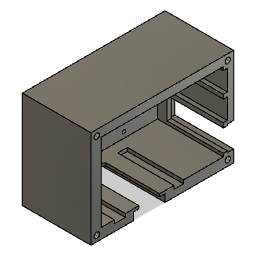
Main Pi Case v10 (Autodesk Fusion 360 design; units mm, degrees)
Autodesk Fusion 360 part; units mm, degrees
sketch "Sketch1" plane through (0, 0, 0) normal (1, 0, 0) x (0, 0, -1)
  line L0 (-44.5, 28) -> (44.5, 28)
  line L1 (44.5, 28) -> (44.5, -28)
  line L2 (44.5, -28) -> (-44.5, -28)
  line L3 (-44.5, -28) -> (-44.5, 28)
  line L4 (-44.5, 28) -> (44.5, -28) construction
  line L5 (44.5, 28) -> (-44.5, -28) construction
  circle A0 centre (-38, 24.5) radius 1.25
  circle A1 centre (-38, -24.5) radius 1.25
  circle A2 centre (20, 25.1038) radius 1.25
  circle A3 centre (20, -23.8962) radius 1.25
  line L6 (-52, 35.5) -> (52, 35.5)
  line L7 (52, 35.5) -> (52, -35.5)
  line L8 (52, -35.5) -> (-52, -35.5)
  line L9 (-52, -35.5) -> (-52, 35.5)
  line L10 (-52, 35.5) -> (52, -35.5) construction
  line L11 (52, 35.5) -> (-52, -35.5) construction
  line L12 (-44.5, 28) -> (-44.5, 29)
  line L13 (-44.5, 29) -> (44.5, 29)
  line L14 (44.5, 29) -> (44.5, 28)
  circle A4 centre (0, 0) radius 13.5
  line L15 (-15, 15) -> (15, 15)
  line L16 (15, 15) -> (15, -15)
  line L17 (15, -15) -> (-15, -15)
  line L18 (-15, -15) -> (-15, 15)
  line L19 (-15, 15) -> (15, -15) construction
  line L20 (15, 15) -> (-15, -15) construction
  circle A5 centre (13, 13) radius 1.5
  circle A6 centre (-13, 13) radius 1.5
  circle A7 centre (-13, -13) radius 1.5
  circle A8 centre (13, -13) radius 1.5
  dimension "d1" = 89
  dimension "d2" = 56
  dimension "d3" = 2.5
  dimension "d4" = 3.5
  dimension "d5" = 6.5
  dimension "d6" = 2.5
  dimension "d7" = 6.5
  dimension "d8" = 49
  dimension "d9" = 2.5
  dimension "d10" = 2.5
  dimension "d11" = 49
  dimension "d12" = 58
  dimension "d13" = 58
  dimension "d16" = 104
  dimension "d17" = 71
  dimension "d86" = 27
  dimension "d87" = 30
  dimension "d88" = 30
  dimension "d89" = 3
  dimension "d90" = 3
  dimension "d91" = 3
  dimension "d92" = 3
  dimension "d93" = 2
  dimension "d94" = 2
  dimension "d95" = 2
  dimension "d96" = 2
  constraint horizontal L0
  constraint perpendicular L0 L1
  constraint parallel L0 L2
  constraint parallel L1 L3
  constraint coincident L4 A4.centre
  constraint coincident L5 A4.centre
  constraint coincident A4.centre origin
  constraint horizontal L6
  constraint perpendicular L6 L7
  constraint parallel L6 L8
  constraint parallel L7 L9
  constraint coincident L10 A4.centre
  constraint coincident L11 A4.centre
  constraint perpendicular L0 L12
  constraint perpendicular L12 L13
  constraint perpendicular L0 L14
  constraint horizontal L15
  constraint perpendicular L15 L16
  constraint parallel L15 L17
  constraint parallel L16 L18
  constraint coincident L19 A4.centre
  constraint coincident L20 A4.centre
  constraint coincident L20 A5.centre
  constraint coincident L19 A6.centre
  constraint coincident L20 A7.centre
  constraint coincident L19 A8.centre
  measures "d1" distance of L1.end L2.end
  measures "d2" distance of L0.end L1.end
  measures "d3" diameter of A0
  measures "d4" distance of L0 A0.centre
  measures "d5" distance of L3 A0.centre
  measures "d6" diameter of A1
  measures "d7" distance of L3 A1.centre
  measures "d8" distance of A0.centre A1.centre
  measures "d9" diameter of A2 A2.centre
  measures "d10" diameter of A3 A2.centre
  measures "d11" vertical distance of A2.centre A3.centre
  measures "d12" horizontal distance of A0.centre A2.centre
  measures "d13" horizontal distance of A1.centre A3.centre
  measures "d16" distance of L7.end L8.end
  measures "d17" distance of L6.end L7.end
  measures "d86" diameter of A4
  measures "d87" distance of L16.end L17.end A2.centre
  measures "d88" distance of L15.end L16.end A2.centre
  measures "d89" diameter of A5
  measures "d90" diameter of A6
  measures "d91" diameter of A7
  measures "d92" diameter of A8
  measures "d93" distance of L16 A8.centre
  measures "d94" distance of L16 A5.centre
  measures "d95" distance of L18 A6.centre
  measures "d96" distance of L18 A7.centre
extrude "Extrude1" add sketch "Sketch1" along normal blind 2 contours L0 L12 L13 L14 | L0 L1 L2 L3 | L15 L16 L17 L18
extrude "Extrude2" add sketch "Sketch1" along normal blind 50 contours L6 L7 L8 L9
sketch "Sketch2" plane through (0, -28, 0) normal (0, 1, 0) x (-1, 0, 0)
  line L0 (-2, -44.5) -> (-2, 44.5)
  line L1 (-2, 44.5) -> (-50, 44.5)
  line L2 (-50, 44.5) -> (-50, -44.5)
  line L3 (-50, -44.5) -> (-2, -44.5)
  line L4 (-9, 34.9) -> (-12, 34.9)
  line L5 (-12, 34.9) -> (-12, 26.9)
  line L6 (-12, 26.9) -> (-9, 26.9)
  line L7 (-9, 26.9) -> (-9, 34.9)
  line L8 (-12, 34.9) -> (-50, 34.9)
  line L9 (-50, 34.9) -> (-50, 26.9)
  line L10 (-50, 26.9) -> (-12, 26.9)
  line L11 (-12, 26.9) -> (-12, 34.9)
  line L12 (-9, 14.4989) -> (-9, 4.4989)
  line L13 (-9, 4.4989) -> (-11.002, 2)
  line L14 (-11.002, 2) -> (-15.002, 2)
  line L15 (-15.002, 2) -> (-15.002, 17)
  line L16 (-15.002, 17) -> (-11.002, 17)
  line L17 (-11.002, 17) -> (-9, 14.4989)
  line L18 (-15.002, 17) -> (-50, 17)
  line L19 (-50, 17) -> (-50, 2)
  line L20 (-50, 2) -> (-15.002, 2)
  line L21 (-15.002, 2) -> (-15.002, 17)
  line L22 (-9, -8.5) -> (-16, -8.5)
  line L23 (-16, -8.5) -> (-16, -15.5)
  line L24 (-16, -15.5) -> (-9, -15.5)
  line L25 (-9, -15.5) -> (-9, -8.5)
  line L26 (-16, -8.5) -> (-50.0121, -8.5)
  line L27 (-50.0121, -8.5) -> (-50.0121, -15.5)
  line L28 (-50.0121, -15.5) -> (-16, -15.5)
  line L29 (-16, -15.5) -> (-16, -8.5)
  dimension "d20" = 3
  dimension "d21" = 8
  dimension "d22" = 9.6
  dimension "d30" = 10
  dimension "d33" = 4
  dimension "d34" = 15
  dimension "d35" = 4
  dimension "d36" = 7
  dimension "d37" = 7
  dimension "d38" = 27.5
  dimension "d39" = 7
  dimension "d40" = 7
  dimension "d41" = 7
  dimension "d42" = 53
  constraint horizontal L4
  constraint vertical L5
  constraint horizontal L6
  constraint vertical L7
  constraint horizontal L8
  constraint vertical L9
  constraint horizontal L10
  constraint vertical L11
  constraint vertical L12
  constraint horizontal L14
  constraint perpendicular L14 L15
  constraint perpendicular L15 L16
  constraint horizontal L18
  constraint vertical L19
  constraint horizontal L20
  constraint vertical L21
  constraint horizontal L22
  constraint vertical L23
  constraint horizontal L24
  constraint vertical L25
  constraint horizontal L26
  constraint vertical L27
  constraint horizontal L28
  constraint vertical L29
  measures "d20" distance of L4.start L4.end
  measures "d21" distance of L4.start L6.end
  measures "d22" distance of L1 L4
  measures "d30" distance of L12.start L12.end
  measures "d33" distance of L13.end L14.end
  measures "d34" distance of L14.end L15.end
  measures "d35" distance of L15.end L16.end
  measures "d36" distance of L0 L7
  measures "d37" distance of L0 L12
  measures "d38" distance of L1 L16
  measures "d39" distance of L22.start L22.end
  measures "d40" distance of L22.start L24.end
  measures "d41" distance of L0 L25
  measures "d42" distance of L1 L22
extrude "Extrude3" cut sketch "Sketch2" against normal blind 2.5 contours L2 L26 L27 L28 | L2 L23 L26 L28 L29 | L2 L5 L8 L9 L10 L11 | L22 L23 L24 L25 L29 | L4 L5 L6 L7 L11 | L2 L15 L18 L19 L20 L21 | L12 L13 L14 L15 L16 L17 L21
sketch "Sketch3" plane through (0, -35.5, 0) normal (0, -1, 0) x (1, 0, 0)
  line L0 (0, 52) -> (0, -52)
  line L1 (0, -52) -> (50, -52)
  line L2 (50, -52) -> (50, 52)
  line L3 (50, 52) -> (0, 52)
  line L4 (19.5, 21) -> (4.5, 21)
  line L5 (4.5, 21) -> (4.5, -2)
  line L6 (4.5, -2) -> (19.5, -2)
  line L7 (19.5, -2) -> (19.5, 21)
  line L8 (19.5, 21) -> (50, 21)
  line L9 (50, 21) -> (50, -2)
  line L10 (50, -2) -> (19.5, -2)
  line L11 (19.5, -2) -> (19.5, 21)
  dimension "d45" = 15
  dimension "d46" = 23
  dimension "d47" = 31
  dimension "d48" = 4.5
  constraint horizontal L4
  constraint vertical L5
  constraint horizontal L6
  constraint vertical L7
  constraint horizontal L8
  constraint vertical L9
  constraint horizontal L10
  constraint vertical L11
  constraint coincident L2 L9.end
  measures "d45" distance of L4.start L4.end
  measures "d46" distance of L4.start L6.end
  measures "d47" distance of L3 L4
  measures "d48" distance of L0 L5
extrude "Extrude4" cut sketch "Sketch3" against normal blind 5.5 contours L2 L7 L8 L9 L10 L11 | L4 L5 L6 L7 L11
sketch "Sketch4" plane through (0, 0, -44.5) normal (0, 0, 1) x (1, 0, 0)
  line L0 (2, 29) -> (2, -28)
  line L1 (2, -28) -> (50, -28)
  line L2 (50, -28) -> (50, 29)
  line L3 (9, -25.75) -> (22.5, -25.75)
  line L4 (22.5, -25.75) -> (22.5, -9.75)
  line L5 (22.5, -9.75) -> (9, -9.75)
  line L6 (9, -9.75) -> (9, -25.75)
  line L7 (25, -6.5) -> (9, -6.5)
  line L8 (9, -6.5) -> (9, 8.5)
  line L9 (9, 8.5) -> (25, 8.5)
  line L10 (25, 8.5) -> (25, -6.5)
  line L11 (25, 11.5) -> (9, 11.5)
  line L12 (9, 11.5) -> (9, 26.5)
  line L13 (9, 26.5) -> (25, 26.5)
  line L14 (25, 26.5) -> (25, 11.5)
  line L15 (25, 26.5) -> (50, 26.5)
  line L16 (50, 26.5) -> (50, 11.5)
  line L17 (50, 11.5) -> (25, 11.5)
  line L18 (25, 11.5) -> (25, 26.5)
  line L19 (25, 8.5) -> (50, 8.5)
  line L20 (50, 8.5) -> (50, -6.5)
  line L21 (50, -6.5) -> (25, -6.5)
  line L22 (25, -6.5) -> (25, 8.5)
  line L23 (22.5, -9.75) -> (50, -9.75)
  line L24 (50, -9.75) -> (50, -25.75)
  line L25 (50, -25.75) -> (22.5, -25.75)
  line L26 (22.5, -25.75) -> (22.5, -9.75)
  line L27 (50, 29) -> (2, 29)
  dimension "d51" = 13.5
  dimension "d52" = 16
  dimension "d53" = 2.25
  dimension "d54" = 7
  dimension "d55" = 16
  dimension "d56" = 15
  dimension "d57" = 7
  dimension "d58" = 21.5
  dimension "d59" = 16
  dimension "d60" = 15
  dimension "d61" = 7
  dimension "d62" = 39.5
  dimension "d65" = 15
  constraint horizontal L3
  constraint vertical L4
  constraint horizontal L5
  constraint vertical L6
  constraint horizontal L7
  constraint vertical L8
  constraint horizontal L9
  constraint vertical L10
  constraint horizontal L11
  constraint vertical L12
  constraint horizontal L13
  constraint vertical L14
  constraint horizontal L15
  constraint vertical L16
  constraint horizontal L17
  constraint vertical L18
  constraint horizontal L19
  constraint vertical L20
  constraint horizontal L21
  constraint vertical L22
  constraint coincident L2 L20.end
  constraint horizontal L23
  constraint vertical L24
  constraint horizontal L25
  constraint vertical L26
  constraint coincident L2 L24.end
  measures "d51" distance of L3.start L3.end
  measures "d52" distance of L3.start L5.end
  measures "d53" distance of L1 L3
  measures "d54" distance of L0 L6
  measures "d55" distance of L7.start L7.end
  measures "d56" distance of L7.start L9.end
  measures "d57" distance of L0 L8
  measures "d58" distance of L1 L7
  measures "d59" distance of L11.start L11.end
  measures "d60" distance of L11.start L13.end
  measures "d61" distance of L0 L12
  measures "d62" distance of L1 L11
  measures "d65" distance of L13.end L11.start
extrude "Extrude5" cut sketch "Sketch4" against normal blind 3 contours L2 L14 L15 L16 L17 L18 | L2 L4 L23 L24 L25 L26 | L11 L12 L13 L14 L18 | L3 L4 L5 L6 L26 | L2 L10 L19 L20 L21 L22 | L7 L8 L9 L10 L22
sketch "Sketch5" plane through (0, 0, -52) normal (0, 0, -1) x (-1, 0, 0)
  line L0 (0, -35.5) -> (0, 35.5)
  line L1 (0, 35.5) -> (-50, 35.5)
  line L2 (-50, 35.5) -> (-50, -35.5)
  line L3 (-50, -35.5) -> (0, -35.5)
  line L4 (-7, -26.75) -> (-23, -26.75)
  line L5 (-23, -26.75) -> (-23, -8.75)
  line L6 (-23, -8.75) -> (-7, -8.75)
  line L7 (-7, -8.75) -> (-7, -26.75)
  line L8 (-23, -8.75) -> (-50, -8.75)
  line L9 (-50, -8.75) -> (-50, -26.75)
  line L10 (-50, -26.75) -> (-23, -26.75)
  line L11 (-23, -26.75) -> (-23, -8.75)
  dimension "d66" = 16
  dimension "d67" = 18
  dimension "d68" = 8.75
  dimension "d69" = 7
  constraint horizontal L4
  constraint vertical L5
  constraint horizontal L6
  constraint vertical L7
  constraint horizontal L8
  constraint vertical L9
  constraint horizontal L10
  constraint vertical L11
  constraint coincident L2 L9.end
  measures "d66" distance of L4.start L4.end
  measures "d67" distance of L4.start L6.end
  measures "d68" distance of L3 L4
  measures "d69" distance of L0 L7
extrude "Extrude6" cut sketch "Sketch5" against normal blind 4.5 contours L2 L5 L8 L9 L10 L11 | L4 L5 L6 L7 L11
sketch "Sketch6" plane through (50, 0, 0) normal (1, 0, 0) x (0, 0, -1)
  line L0 (47.5, -8.75) -> (52, -8.75)
  line L1 (52, -8.75) -> (52, 35.5)
  line L2 (52, 35.5) -> (-52, 35.5)
  line L3 (-52, 35.5) -> (-52, -35.5)
  line L4 (-52, -35.5) -> (-21, -35.5)
  line L5 (-21, -35.5) -> (-21, -30)
  line L6 (-21, -30) -> (-17, -30)
  line L7 (-17, -30) -> (-17, -28)
  line L8 (-17, -28) -> (-26.9, -28)
  line L9 (-26.9, -28) -> (-26.9, -30.5)
  line L10 (-26.9, -30.5) -> (-34.9, -30.5)
  line L11 (-34.9, -30.5) -> (-34.9, -28)
  line L12 (-34.9, -28) -> (-44.5, -28)
  line L13 (-44.5, -28) -> (-44.5, 29)
  line L14 (44.5, 29) -> (44.5, 26.5)
  line L15 (44.5, 26.5) -> (47.5, 26.5)
  line L16 (47.5, 26.5) -> (47.5, 11.5)
  line L17 (47.5, 11.5) -> (44.5, 11.5)
  line L18 (44.5, 11.5) -> (44.5, 8.5)
  line L19 (44.5, 8.5) -> (47.5, 8.5)
  line L20 (47.5, 8.5) -> (47.5, -6.5)
  line L21 (47.5, -6.5) -> (44.5, -6.5)
  line L22 (44.5, -6.5) -> (44.5, -9.75)
  line L23 (44.5, -9.75) -> (47.5, -9.75)
  line L24 (47.5, -9.75) -> (47.5, -8.75)
  circle A0 centre (-47.75, 31.25) radius 2
  circle A1 centre (-47.75, -31.25) radius 2
  circle A2 centre (47.75, 31.25) radius 2
  circle A3 centre (47.75, -31.25) radius 2
  line L25 (52, -35.5) -> (52, -26.75)
  line L26 (2, -35.5) -> (52, -35.5)
  line L27 (-44.5, 29) -> (44.5, 29)
  dimension "d72" = 4
  dimension "d73" = 4
  dimension "d74" = 4
  dimension "d75" = 4
  dimension "d76" = 4.25
  dimension "d77" = 4.25
  dimension "d78" = 4.25
  dimension "d79" = 4.25
  dimension "d80" = 4.25
  dimension "d81" = 4.25
  dimension "d82" = 4.25
  dimension "d83" = 4.25
  measures "d72" diameter of A0
  measures "d73" diameter of A1
  measures "d74" diameter of A2
  measures "d75" diameter of A3
  measures "d76" distance of L3 A1.centre
  measures "d77" distance of L4 A1.centre
  measures "d78" distance of L2 A0.centre
  measures "d79" distance of L3 A0.centre
  measures "d80" distance of L2 A2.centre
  measures "d81" distance of L1 A2.centre
  measures "d82" distance of A3.centre L25
  measures "d83" distance of A3.centre L26
extrude "Extrude7" cut sketch "Sketch6" against normal blind 4.75 contours A0 | A1 | A2 | A3
